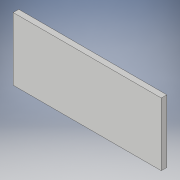
# Autodesk Inventor part: Bottom
Saved by Autodesk Inventor 2018 (Build 220112000, 112)
## iProperties
Created: 2018-04-18
Part Number: Bottom
Material: Generic
Document SubType Name: Modeling
Designer: trent
Density: 1 g/cm^3
Appearance: Default
Author: trent
Autodesk Inventor part; units mm, degrees
ref_plane "YZ Plane" through (0, 0, 0) normal (1, 0, 0) x (0, 1, 0)
ref_plane "XZ Plane" through (0, 0, 0) normal (0, 1, 0) x (-1, 0, 0)
ref_plane "XY Plane" through (0, 0, 0) normal (0, 0, 1) x (1, 0, 0)
sketch "Sketch1" plane through (0, 0, 0) normal (0, 0, 1) x (1, 0, 0)
  line L0 (0, 0) -> (127, 0)
  line L1 (127, 0) -> (127, 53.975)
  line L2 (127, 53.975) -> (0, 53.975)
  line L3 (0, 53.975) -> (0, 0)
  dimension "d0" = 127
  dimension "d1" = 53.975
  constraints: 8 end point, 2 parallel, 1 horizontal, 1 perpendicular
  measures "d0" distance of L2.end L1.end
  measures "d1" distance of L1.end L0.end
extrude "Extrusion1" add sketch "Sketch1" along normal blind 4.7625
body "Solid1"
